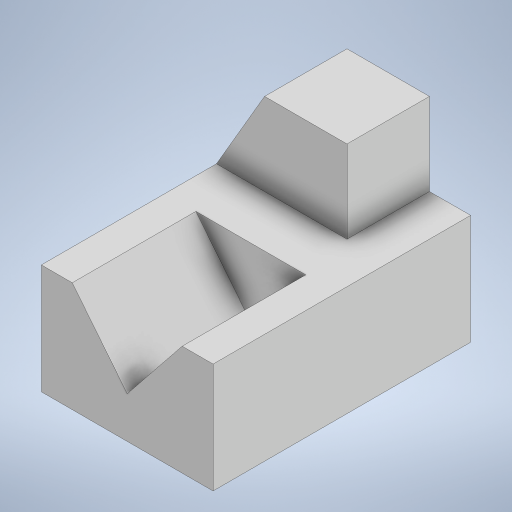
# Autodesk Inventor part: 6 - Part 1
Saved by Autodesk Inventor 2024 (Build 280153000, 153)
## iProperties
Created: 2024-04-21
Part Number: 6 - Part 1
Material: Generic
Document SubType Name: Modeling
Designer: Ricsi
Density: 1 g/cm^3
Appearance: Default
Author: Ricsi
Autodesk Inventor part; units mm, degrees
ref_plane "YZ Plane" through (0, 0, 0) normal (1, 0, 0) x (0, 1, 0)
ref_plane "XZ Plane" through (0, 0, 0) normal (0, 1, 0) x (-1, 0, 0)
ref_plane "XY Plane" through (0, 0, 0) normal (0, 0, 1) x (1, 0, 0)
sketch "Sketch1" plane through (0, 0, 0) normal (0, 1, 0) x (-1, 0, 0)
  line L0 (11.9058, 27.912) -> (-38.0942, 27.912)
  line L1 (-38.0942, 27.912) -> (-38.0942, -47.088)
  line L2 (-38.0942, -47.088) -> (11.9058, -47.088)
  line L3 (11.9058, -47.088) -> (11.9058, 27.912)
  point P0 (0, 0)
  dimension "d0" = 50
  dimension "d1" = 75
  constraints: 8 end point, 2 parallel, 1 horizontal, 1 perpendicular
  measures "d0" distance of L2.end L1.end
  measures "d1" distance of L1.end L0.end
extrude "Extrusion1" add sketch "Sketch1" along normal blind 32
sketch "Sketch2" plane through (-11.9058, 0, 27.912) normal (0, 0, 1) x (1, 0, 0)
  line L0 (0, 0) -> (25, 0)
  line L1 (0, 32) -> (9, 32)
  line L2 (41, 32) -> (25, 12)
  line L3 (9, 32) -> (25, 12)
  line L4 (9, 32) -> (41, 32)
  line L5 (50, 32) -> (0, 32) projected
  line L6 (0, 0) -> (0, 32) projected
  point P0 (11.9058, 0)
  dimension "d8" = 38.66
  constraints: 10 end point, 1 collinear
  measures "d8" angle of L6 L3
extrude "Extrusion2" cut sketch "Sketch2" against normal blind 36
sketch "Sketch3" plane through (0, 32, 0) normal (0, 1, 0) x (1, 0, 0)
  line L0 (-11.9058, 47.088) -> (-11.9058, -27.912) projected
  line L1 (-11.9058, 47.088) -> (-11.9058, 23.088)
  line L2 (38.0942, 47.088) -> (26.0942, 47.088)
  line L3 (-11.9058, 47.088) -> (26.0942, 47.088)
  line L4 (38.0942, 47.088) -> (-11.9058, 47.088) projected
  line L5 (-11.9058, 23.088) -> (26.0942, 23.088)
  line L6 (26.0942, 23.088) -> (26.0942, 47.088)
  point P0 (0, 0)
  dimension "d11" = 24
  dimension "d13" = 38
  dimension "d14" = 38
  constraints: 10 end point, 1 collinear, 1 horizontal, 1 point on line
  measures "d11" distance of L0.start L1.end
  measures "d13" distance of L0.start L2.end
  measures "d14" distance of L1.end L5.end
extrude "Extrusion3" add sketch "Sketch3" along normal blind 24
sketch "Sketch4" plane through (-11.9058, 32, -23.088) normal (0, 0, 1) x (1, 0, 0)
  line L0 (0, -32) -> (0, 24) projected
  line L1 (0, 24) -> (14, 24)
  line L2 (0, 24) -> (38, 24) projected
  line L3 (0, 0) -> (9, 0) projected
  line L4 (14, 24) -> (0, 0)
  line L5 (0, 0) -> (0, 24)
  point P0 (11.9058, -32)
  dimension "d17" = 14
  constraints: 6 end point, 1 collinear, 1 point on line
  measures "d17" distance of L0.end L1.end
extrude "Extrusion4" cut sketch "Sketch4" against normal blind 24
body "Solid1"
